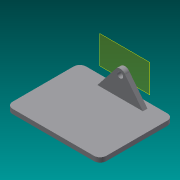
# Autodesk Inventor part: headtilt-base
Saved by Autodesk Inventor 2013 SP2 (Build 170200200, 200)
## iProperties
Created: 2014-11-25
Part Number: headtilt-base
Material: Generic
Document SubType Name: Modeling
Designer: Master
Density: 1 g/cm^3
Author: Master
Autodesk Inventor part; units mm, degrees
ref_plane "YZ Plane" through (0, 0, 0) normal (1, 0, 0) x (0, 1, 0)
ref_plane "XZ Plane" through (0, 0, 0) normal (0, 1, 0) x (-1, 0, 0)
ref_plane "XY Plane" through (0, 0, 0) normal (0, 0, 1) x (1, 0, 0)
ref_plane "Work Plane1" through (0, 0, 0) normal (0, 0, 1) x (1, 0, 0)
sketch "Sketch1" plane through (0, 0, 0) normal (0, 0, 1) x (1, 0, 0)
  circle A0 centre (0, -6.2841) radius 1.4986 projected
  arc A1 (-2.5077, -7.7319) -> (2.5077, -7.7319) centre (0, -6.2841) ccw projected
  line L0 (-2.5077, -7.7319) -> (-11.746, 4.0347) projected
  line L1 (11.746, 4.0347) -> (-11.746, 4.0347) projected
  line L2 (11.746, 4.0347) -> (2.5077, -7.7319) projected
  circle A2 centre (0, -6.2841) radius 1.4986
  line L3 (-11.746, 4.0347) -> (-3.6444, -6.2841)
  line L4 (3.6444, -6.2841) -> (11.746, 4.0347)
  line L5 (11.746, 4.0347) -> (-11.746, 4.0347)
  line L6 (2.5077, -4.8363) -> (11.7464, -16.6034)
  line L7 (-2.5077, -4.8363) -> (-11.7464, -16.6034)
  line L8 (-11.7464, -16.6034) -> (11.7464, -16.6034)
  arc A3 (2.5077, -4.8363) -> (-2.5077, -4.8363) centre (0, -6.2841) ccw
  point P0 (0, 0)
  dimension "d0" = 14.9606
  dimension "d1" = 14.9606
  constraints: 13 end point, 2 centre point, 2 collinear, 2 parallel, 2 point on circle, 2 point on line, 1 coincident, 1 concentric
  measures "d0" distance of L6.start L6.end
  measures "d1" distance of L7.start L7.end
extrude "Extrusion1" add sketch "Sketch1" along normal blind 2.3813 contours L0 L7 A3 L6 L2 A1 | A1 L2 L6 L8 L7 L0
sketch "Sketch2" plane through (-11.7464, -16.6034, 0) normal (0, -1, 0) x (1, 0, 0)
  line L0 (5.9964, 35) -> (26.2464, 35) projected
  line L1 (20.4964, -2.75) -> (29.2464, -2.75) projected
  line L2 (-7.5036, -3) -> (1.4964, -3) projected
  line L3 (-14.5036, 16.05) -> (-14.5036, 26.8) projected
  line L4 (33.9964, 15.95) -> (33.9964, 5) projected
  line L5 (-14.5036, 26.8) -> (-14.5036, -3)
  line L6 (-14.5036, -3) -> (33.9964, -3)
  line L7 (33.9964, -3) -> (33.9964, 35)
  line L8 (33.9964, 35) -> (-14.5036, 35)
  line L9 (-14.5036, -3) -> (-14.5036, 35)
  point P0 (11.7464, 0)
  constraints: 10 end point, 4 perpendicular, 1 parallel
extrude "Extrusion2" add sketch "Sketch2" along normal blind 2.3813
fillet "Fillet1" radius 3.175 1 edges at (-26.25, -17.794, -3)
fillet "Fillet2" radius 3.175 1 edges at (-26.25, -17.794, 35)
fillet "Fillet3" radius 3.175 1 edges at (22.25, -17.794, 35)
fillet "Fillet4" radius 3.175 1 edges at (22.25, -17.794, -3)
body "Solid1"
